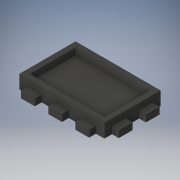
# Autodesk Inventor part: bottom
Saved by Autodesk Inventor 2019 (Build 230136000, 136)
## iProperties
Created: 2018-06-06
Part Number: bottom
Material: PBT Plastic Black
Document SubType Name: Modeling
Designer: stra92745
Density: 1.31 g/cm^3
Appearance: Smooth - White
Author: stra92745
Autodesk Inventor part; units mm, degrees
ref_plane "YZ Plane" through (0, 0, 0) normal (1, 0, 0) x (0, 1, 0)
ref_plane "XZ Plane" through (0, 0, 0) normal (0, 1, 0) x (-1, 0, 0)
ref_plane "XY Plane" through (0, 0, 0) normal (0, 0, 1) x (1, 0, 0)
sketch "Sketch1" plane through (0, 0, 0) normal (0, 1, 0) x (-1, 0, 0)
  line L0 (0, 0) -> (-58, 0)
  line L1 (-58, 0) -> (-58, -41)
  line L2 (-58, -41) -> (0, -41)
  line L3 (0, -41) -> (0, 0)
  dimension "d0" = 58
  dimension "d1" = 41
  constraints: 8 end point, 2 parallel, 1 horizontal, 1 perpendicular
  measures "d0" distance of L2.end L1.end
  measures "d1" distance of L1.end L0.end
extrude "Extrusion1" add sketch "Sketch1" along normal blind 4
sketch "Sketch2" plane through (0, 4, 0) normal (0, 1, 0) x (1, 0, 0)
  line L0 (0, 0) -> (58, 0) projected
  line L1 (58, 0) -> (58, 41) projected
  line L2 (58, 41) -> (0, 41) projected
  line L3 (0, 41) -> (0, 0) projected
  line L4 (4, 37) -> (54, 37)
  line L5 (54, 37) -> (54, 4)
  line L6 (54, 4) -> (4, 4)
  line L7 (4, 4) -> (4, 37)
  line L8 (51, 34) -> (7, 34)
  line L9 (7, 34) -> (7, 7)
  line L10 (7, 7) -> (51, 7)
  line L11 (51, 7) -> (51, 34)
  dimension "d4" = 4
  dimension "d5" = 3
  constraints: 16 end point, 6 other
  measures "d4" distance between parallel lines of L2 L4
  measures "d5" distance between parallel lines of L4 L8
extrude "Extrusion2" add sketch "Sketch2" along normal blind 4 contours L4 L5 L6 L7
sketch "Sketch3" plane through (0, 4, 0) normal (0, 1, 0) x (1, 0, 0)
  line L0 (0, 0) -> (58, 0) construction
  line L1 (58, 0) -> (58, 41) construction
  line L2 (58, 41) -> (0, 41) construction
  line L3 (0, 41) -> (0, 0) construction
  line L4 (54, 37) -> (54, 4) construction
  line L5 (54, 4) -> (4, 4) construction
  line L6 (4, 4) -> (4, 37) construction
  line L7 (4, 37) -> (54, 37) construction
  line L8 (58, 41) -> (0, 41) construction
  line L9 (29, 41) -> (29, 0) construction
  line L10 (0, 41) -> (0, 0) construction
  line L11 (0, 20.5) -> (58, 20.5) construction
  line L12 (58, 0) -> (58, 41) construction
  line L13 (4, 37) -> (4, 4) projected
  line L14 (4, 8.5) -> (0, 8.5)
  line L15 (0, 8.5) -> (0, 0)
  line L16 (0, 0) -> (9, 0)
  line L17 (0, 0) -> (58, 0) projected
  line L18 (9, 0) -> (9, 4)
  line L19 (54, 4) -> (4, 4) projected
  line L20 (9, 4) -> (4, 4)
  line L21 (4, 8.5) -> (4, 4)
  line L22 (17, 0) -> (17, 4)
  line L23 (17, 0) -> (25, 0)
  line L24 (25, 0) -> (25, 4)
  line L25 (25, 4) -> (17, 4)
  line L26 (0, 16.5) -> (4, 16.5)
  line L27 (4, 16.5) -> (4, 20.5)
  line L28 (0, 20.5) -> (0, 16.5)
  line L29 (4, 32.5) -> (0, 32.5)
  line L30 (0, 32.5) -> (0, 41)
  line L31 (0, 41) -> (9, 41)
  line L32 (9, 41) -> (9, 37)
  line L33 (9, 37) -> (4, 37)
  line L34 (4, 32.5) -> (4, 37)
  line L35 (17, 41) -> (17, 37)
  line L36 (17, 41) -> (25, 41)
  line L37 (25, 41) -> (25, 37)
  line L38 (25, 37) -> (17, 37)
  line L39 (0, 24.5) -> (4, 24.5)
  line L40 (4, 24.5) -> (4, 20.5)
  line L41 (0, 20.5) -> (0, 24.5)
  line L42 (58, 41) -> (58, 0) construction
  line L43 (54, 4) -> (54, 37) construction
  line L44 (58, 41) -> (58, 0) construction
  line L45 (54, 37) -> (54, 4)
  line L46 (54, 8.5) -> (58, 8.5)
  line L47 (58, 8.5) -> (58, 0)
  line L48 (58, 0) -> (49, 0)
  line L49 (49, 0) -> (49, 4)
  line L50 (49, 4) -> (54, 4)
  line L51 (54, 8.5) -> (54, 4)
  line L52 (41, 0) -> (41, 4)
  line L53 (41, 0) -> (33, 0)
  line L54 (33, 0) -> (33, 4)
  line L55 (33, 4) -> (41, 4)
  line L56 (58, 16.5) -> (54, 16.5)
  line L57 (54, 16.5) -> (54, 20.5)
  line L58 (58, 20.5) -> (58, 16.5)
  line L59 (41, 41) -> (33, 41)
  line L60 (33, 41) -> (33, 37)
  line L61 (33, 37) -> (41, 37)
  line L62 (54, 32.5) -> (54, 37)
  line L63 (54, 24.5) -> (54, 20.5)
  line L64 (54, 32.5) -> (58, 32.5)
  line L65 (58, 32.5) -> (58, 41)
  line L66 (58, 24.5) -> (54, 24.5)
  line L67 (58, 20.5) -> (58, 24.5)
  line L68 (49, 41) -> (49, 37)
  line L69 (49, 37) -> (54, 37)
  line L70 (58, 41) -> (49, 41)
  line L71 (41, 41) -> (41, 37)
  dimension "d8" = 8
  dimension "d9" = 8
  dimension "d10" = 4
  dimension "d13" = 4
  dimension "d14" = 8
  constraints: 116 end point, 38 symmetric about line, 14 point on line, 6 perpendicular, 5 midpoint, 2 collinear, 1 horizontal, 1 parallel
  measures "d8" distance of L22.start L23.end
  measures "d9" distance between parallel lines of L22 L18
  measures "d10" distance between parallel lines of L9 L24
  measures "d13" distance of L11.start L26.start
  measures "d14" distance between parallel lines of L14 L26
extrude "Extrusion3" cut sketch "Sketch3" against normal up to surface (4 mm away) contours L13 L29 L30 L31 L32 L33 | L13 L26 L28 L41 L39 | L13 L19 L18 L16 L15 L14 | L19 L24 L17 L22 | L19 L52 L17 L54 | L19 L45 L46 L47 L17 L49 | L36 L37 L38 L35 | L69 L68 L70 L65 L64 L45 | L66 L67 L58 L56 L45 | L71 L61 L60 L59
body "Solid1"
